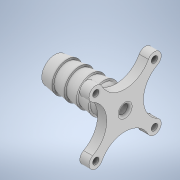
# Autodesk Inventor part: NozzleAdapter
Saved by Autodesk Inventor 2020 (Build 240168000, 168)
## iProperties
Created: 2019-04-28
Part Number: NozzleAdapter
Material: Generic
Document SubType Name: Modeling
Designer: Connor
Density: 1 g/cm^3
Appearance: Default
Author: Connor
Autodesk Inventor part; units mm, degrees
ref_plane "YZ Plane" through (0, 0, 0) normal (1, 0, 0) x (0, 1, 0)
ref_plane "XZ Plane" through (0, 0, 0) normal (0, 1, 0) x (-1, 0, 0)
ref_plane "XY Plane" through (0, 0, 0) normal (0, 0, 1) x (1, 0, 0)
sketch "Sketch3" plane through (0, 0, 0) normal (0, 0, 1) x (1, 0, 0)
  line L0 (0, 0) -> (0, 4.572)
  line L1 (0, 4.572) -> (4.2333, 5.2324)
  line L2 (0, 0) -> (21.1667, 0)
  line L3 (4.2333, 5.2324) -> (4.2333, 4.572)
  line L4 (4.2333, 4.572) -> (8.4667, 5.2324)
  line L5 (8.4667, 5.2324) -> (8.4667, 4.572)
  line L6 (8.4667, 4.572) -> (12.7, 5.2324)
  line L7 (12.7, 5.2324) -> (12.7, 4.572)
  line L8 (12.7, 4.572) -> (16.9333, 5.2324)
  line L9 (16.9333, 5.2324) -> (16.9333, 4.572)
  line L10 (16.9333, 4.572) -> (21.1667, 5.2324)
  line L11 (21.1667, 5.2324) -> (21.1667, 0)
  line L12 (21.1667, 0) -> (24.3417, 0)
  line L13 (24.3417, 0) -> (24.3417, 6.35)
  line L14 (24.3417, 6.35) -> (21.1667, 6.35)
  line L15 (21.1667, 6.35) -> (21.1667, 0)
  dimension "d4" = 4.572
  dimension "d6" = 5.2324
  dimension "d7" = 4.2333
  dimension "d8" = 3.175
  dimension "d9" = 6.35
  constraints: 32 end point, 14 parallel, 3 horizontal alignment, 3 vertical, 2 horizontal, 1 perpendicular
  measures "d4" distance of L0.start L0.end
  measures "d6" distance from line of L2 L1.end
  measures "d7" horizontal distance of L1.end L0.end
  measures "d8" distance of L14.end L13.end
  measures "d9" distance of L12.end L13.end
revolve "Revolution1" add sketch "Sketch3" angle 360 about axis through (0, 0, 0) along (1, 0, 0)
sketch "Sketch4" plane through (0, 0, 0) normal (-1, 0, 0) x (0, 0, 1)
  circle A0 centre (0, 0) radius 3.6322
  dimension "d11" = 7.2644
  constraints: 1 centre point, 1 coincident
  measures "d11" diameter of A0
sketch "Sketch5" plane through (24.3417, 0, 0) normal (1, 0, 0) x (0, 0, -1)
  circle A0 centre (0, 0) radius 1.5875
  dimension "d15" = 3.175
  constraints: 1 centre point, 1 coincident
  measures "d15" diameter of A0
loft "Loft1" cut profiles "Sketch4", "Sketch5"
fillet "Fillet2" radius 0.7937 1 edges at (0, 0, -3.6322)
sketch "Sketch6" plane through (24.3417, 0, 0) normal (1, 0, 0) x (0, 0, -1)
  circle A0 centre (0, 0) radius 6.35 projected
  line L0 (-10.16, 10.16) -> (10.16, 10.16) construction
  line L1 (10.16, 10.16) -> (10.16, -10.16) construction
  line L2 (10.16, -10.16) -> (-10.16, -10.16) construction
  line L3 (-10.16, -10.16) -> (-10.16, 10.16) construction
  line L4 (-10.16, 10.16) -> (10.16, -10.16) construction
  line L5 (-10.16, -10.16) -> (10.16, 10.16) construction
  circle A1 centre (-10.16, 10.16) radius 1.1
  circle A2 centre (10.16, 10.16) radius 1.1
  circle A3 centre (10.16, -10.16) radius 1.1
  circle A4 centre (-10.16, -10.16) radius 1.1
  circle A5 centre (-10.16, 10.16) radius 2.37
  circle A6 centre (10.16, 10.16) radius 2.37
  circle A7 centre (10.16, -10.16) radius 2.37
  circle A8 centre (-10.16, -10.16) radius 2.37
  arc A9 (-6.35, 0) -> (-11.2499, 8.0555) centre (-15.4216, 0) ccw
  arc A10 (-8.0555, 11.2499) -> (0, 6.35) centre (0, 15.4216) ccw
  arc A11 (0, -6.35) -> (-8.0555, -11.2499) centre (0, -15.4216) ccw
  arc A12 (-11.2499, -8.0555) -> (-6.35, 0) centre (-15.4216, 0) ccw
  arc A13 (6.35, 0) -> (11.2499, -8.0555) centre (15.4216, 0) ccw
  arc A14 (8.0555, -11.2499) -> (0, -6.35) centre (0, -15.4216) ccw
  arc A15 (0, 6.35) -> (8.0555, 11.2499) centre (0, 15.4216) ccw
  arc A16 (11.2499, 8.0555) -> (6.35, 0) centre (15.4216, 0) ccw
  point P0 (0, 0)
  point P1 (6.35, 0)
  point P2 (6.35, 0)
  point P3 (6.35, 0)
  point P4 (8.0555, 11.2499)
  point P5 (0, 6.35)
  point P6 (0, 6.35)
  point P7 (0, -6.35)
  point P8 (0, -6.35)
  point P9 (0, -6.35)
  point P10 (8.0555, -11.2499)
  point P11 (11.2499, -8.0555)
  point P12 (-6.35, 0)
  point P13 (-6.35, 0)
  point P14 (-11.2499, -8.0555)
  point P15 (-8.0555, -11.2499)
  dimension "d21" = 20.32
  dimension "d22" = 2.2
  dimension "d23" = 1.27
  dimension "d26" = 360
  constraints: 20 point on circle, 16 centre point, 12 end point, 6 equal radius, 5 coincident, 4 tangent, 3 perpendicular, 2 parallel, 1 horizontal, 1 horizontal alignment, 1 midpoint, 1 vertical alignment, 33 other
  measures "d21" distance of L0.start L0.end
  measures "d22" diameter of A1
  measures "d23" radial gap between concentric circles of A1 A5
extrude "Extrusion3" add sketch "Sketch6" against normal blind 3.175 contours A13 A7 A14 A0 | A0 A15 A6 A16 | A0 A9 A5 A10 | A11 A8 A12 A0 | A7 | A6 | A5 | A8
fillet "Fillet3" radius 0.7937 1 edges at (24.3417, 0, -1.5875)
body "Solid2"
